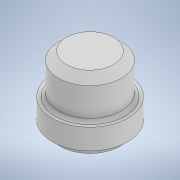
# Autodesk Inventor part: 68. Стопор втулки
Saved by Autodesk Inventor 2021 (Build 250183000, 183)
## iProperties
Created: 2021-03-11
Part Number: 68. Стопор втулки
Material: Типовые
Document SubType Name: Modeling
Designer: Данил
Density: 1 g/cm^3
Appearance: По умолчанию
Author: Данил
Autodesk Inventor part; units mm, degrees
ref_plane "YZ Plane" through (0, 0, 0) normal (1, 0, 0) x (0, 1, 0)
ref_plane "XZ Plane" through (0, 0, 0) normal (0, 1, 0) x (-1, 0, 0)
ref_plane "XY Plane" through (0, 0, 0) normal (0, 0, 1) x (1, 0, 0)
sketch "Эскиз1" plane through (0, 0, 0) normal (0, 0, 1) x (1, 0, 0)
  line L0 (0, 2.15) -> (0, -2.15)
  line L1 (0, -2.15) -> (1.9, -2.15)
  line L2 (2.4, -1.65) -> (2.4, -0.35)
  line L3 (2.4, -0.35) -> (2.2, -0.35)
  line L4 (2, -0.15) -> (2, 1.65)
  line L5 (1.5, 2.15) -> (0, 2.15)
  line L6 (2.4, -1.65) -> (1.9, -2.15)
  line L7 (2, 1.65) -> (1.5, 2.15)
  arc A0 (2, -0.15) -> (2.2, -0.35) centre (2.2, -0.15) ccw
  point P0 (0, 0)
  point P1 (0, 0)
  point P2 (2.4, -2.15)
  point P3 (2, 2.15)
  dimension "d0" = 4.3
  dimension "d1" = 4.8
  dimension "d2" = 4
  dimension "d3" = 1.8
  dimension "d4" = 0.5
  dimension "d5" = 45
  dimension "d6" = 0.5
  dimension "d7" = 45
  dimension "d8" = 0.2
  constraints: 16 end point, 4 perpendicular, 4 point on line, 2 point on circle, 2 tangent, 1 centre point, 1 coincident, 1 horizontal, 1 midpoint, 1 vertical
  measures "d0" distance of L0.start L0.end
  measures "d1" diameter of L2 L0
  measures "d2" diameter of L4 L0
  measures "d3" distance between parallel lines of L1 L3
  measures "d4" distance of L2.start point (2.4, -2.15)
  measures "d5" angle of L2 L6
  measures "d6" distance of L4.end point (2, 2.15)
  measures "d7" angle of L4 L7
  measures "d8" radius of A0
revolve "Вращение1" add sketch "Эскиз1" angle 360 about axis through (0, 2.15, 0) along (0, -1, 0)
equation "\"d6\" = d4"
equation "\"d7\" = d5"
